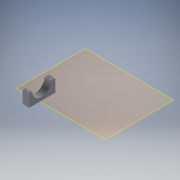
# Autodesk Inventor part: 03_Tubeholder_bottom
Saved by Autodesk Inventor 2016 (Build 200138000, 138)
## iProperties
Created: 2016-09-10
Part Number: 03_Tubeholder_bottom
Material: Generisch
Document SubType Name: Modeling
Designer: Bene
Density: 1 g/cm^3
Appearance: Vorgabe
Author: Bene
Autodesk Inventor part; units mm, degrees
ref_plane "YZ Plane" through (0, 0, 0) normal (1, 0, 0) x (0, 1, 0)
ref_plane "XZ Plane" through (0, 0, 0) normal (0, 1, 0) x (-1, 0, 0)
ref_plane "XY Plane" through (0, 0, 0) normal (0, 0, 1) x (1, 0, 0)
ref_plane "Arbeitsebene1" through (0, 0, 0) normal (0, 0, 1) x (1, 0, 0)
sketch "Skizze1" plane through (0, 0, 0) normal (0, 0, 1) x (1, 0, 0)
  arc A0 (61.9377, 58.8639) -> (58.9377, 61.8639) centre (58.9377, 58.8639) ccw projected
  line L0 (61.9377, 58.8639) -> (61.9377, -61.1361) projected
  arc A1 (58.9377, -64.1361) -> (61.9377, -61.1361) centre (58.9377, -61.1361) ccw projected
  line L1 (58.9377, -64.1361) -> (-54.0623, -64.1361) projected
  arc A2 (-57.0623, -61.1361) -> (-54.0623, -64.1361) centre (-54.0623, -61.1361) ccw projected
  line L2 (-57.0623, -61.1361) -> (-57.0623, -9.9527) projected
  arc A3 (-57.0623, -9.9527) -> (-59.5169, -7.0028) centre (-60.0623, -9.9527) ccw projected
  arc A4 (-66.0623, 0.8639) -> (-59.5169, -7.0028) centre (-58.0623, 0.8639) ccw projected
  line L3 (-66.0623, 0.8639) -> (-66.0623, 58.8639) projected
  arc A5 (-63.0623, 61.8639) -> (-66.0623, 58.8639) centre (-63.0623, 58.8639) ccw projected
  line L4 (-63.0623, 61.8639) -> (58.9377, 61.8639) projected
  line L5 (-66.0182, -50.1361) -> (-47.5182, -50.1361) construction
  line L6 (-66.0182, -25.1361) -> (-47.5182, -25.1361) construction
  line L7 (20.9818, -51.6361) -> (-61.0182, -51.6361) construction
  line L8 (20.9818, -23.6361) -> (-61.0182, -23.6361) construction
  line L9 (-41.5623, -15.514) -> (-44.5623, -15.514) construction
  line L10 (-44.5623, -15.514) -> (-44.5623, -55.514) construction
  line L11 (-44.5623, -55.514) -> (-41.5623, -55.514) construction
  line L12 (-41.5623, -55.514) -> (-41.5623, -15.514) construction
  line L13 (-34.5623, -16.7736) -> (-44.5623, -16.7736)
  line L14 (-44.5623, -16.7736) -> (-44.5623, -56.7736)
  line L15 (-44.5623, -56.7736) -> (-34.5623, -56.7736)
  line L16 (-34.5623, -56.7736) -> (-34.5623, -16.7736)
  circle A6 centre (-48.0623, -46.1361) radius 4 projected
  circle A7 centre (-41.5623, -19.6361) radius 2.5 projected
  circle A8 centre (-41.5623, -53.1361) radius 2.5 projected
  ellipse E0 centre (-61.0181, -37.6361) end of major axis (-61.0181, -23.6361) minor radius 0.0095 projected
  ellipse E1 centre (-66.0181, -37.6361) end of major axis (-66.0181, -50.1361) minor radius 0.0085 projected
  point P0 (0, 0)
  dimension "d0" = 3
  dimension "d1" = 40
  dimension "d2" = 40
  dimension "d3" = 10
  dimension "d9" = 6.8625
  dimension "d10" = 8.1221
  dimension "d11" = 55.5442
  constraints: 24 end point, 6 horizontal, 4 parallel, 2 perpendicular, 1 point on line, 6 other
  measures "d0" distance of L11.end L10.end
  measures "d1" distance of L10.end L9.end
  measures "d2" distance of L14.end L13.end
  measures "d3" distance between parallel lines of L10 L16
  measures "d9" distance between parallel lines of L8 L13
  measures "d10" distance between parallel lines of L8 L9
  measures "d11" distance from line of L8.start L16
extrude "Extrusion1" add sketch "Skizze1" along normal blind 19 contours L16 L15 L14 A6 L13 | A6 L14 | A7 | A8 picked at (-44.4706, -46.5769)
sketch "Skizze2" plane through (-44.5623, -56.7736, 0) normal (-1, 0, 0) x (0, 0, 1)
  circle A0 centre (19.5, 19.1375) radius 14.5027
  ellipse E0 centre (19.4973, 19.1375) end of major axis (19.4973, 33.1375) minor radius 14 projected
  ellipse E1 centre (19.5232, 19.1375) end of major axis (19.5232, 33.3875) minor radius 14.25 (19.5335, 33.3875) -> (19.5128, 4.8875) ccw projected
  ellipse E2 centre (19.5218, 19.1375) end of major axis (19.5218, 31.8875) minor radius 12.75 (19.5311, 31.8875) -> (19.5125, 6.3875) ccw projected
  point P0 (0, 56.7736)
  dimension "d8" = 0.5
  constraints: 1 centre point, 3 other
extrude "Extrusion2" cut sketch "Skizze2" against normal blind 19 contours A0 | E0
sketch "Skizze3" plane through (0, 0, 19) normal (0, 0, 1) x (1, 0, 0)
  circle A0 centre (-41.5623, -19.6361) radius 1.5 construction
  circle A1 centre (-41.5623, -53.1361) radius 1.5 construction
  circle A2 centre (-41.5623, -19.6361) radius 2
  circle A3 centre (-41.5623, -53.1361) radius 2
  point P0 (0, 0)
  dimension "d12" = 4
  dimension "d13" = 4
  constraints: 2 centre point, 2 coincident
  measures "d12" diameter of A2
  measures "d13" diameter of A3
extrude "Extrusion3" cut sketch "Skizze3" against normal through all
